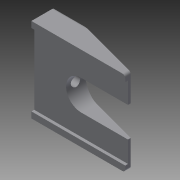
# Autodesk Inventor part: Sliding Block
Saved by Autodesk Inventor 2015 SP2 (Build 190223200, 223)
## iProperties
Created: 2015-12-04
Part Number: Sliding Block
Material: Generic
Document SubType Name: Sheet Metal
Designer: KC-019
Density: 1 g/cm^3
Sheet Metal Rule: Default_mm
Appearance: Default
Author: KC-019
Autodesk Inventor part; units mm, degrees
ref_plane "YZ Plane" through (0, 0, 0) normal (1, 0, 0) x (0, 1, 0)
ref_plane "XZ Plane" through (0, 0, 0) normal (0, 1, 0) x (-1, 0, 0)
ref_plane "XY Plane" through (0, 0, 0) normal (0, 0, 1) x (1, 0, 0)
sketch "Sketch1" plane through (0, 0, 0) normal (0, 1, 0) x (-1, 0, 0)
  arc A0 (0, -16) -> (0, 16) centre (0, 0) ccw
  line L0 (0, 16) -> (-50, 16)
  line L1 (-50, 16) -> (-50, -16)
  line L2 (-50, -16) -> (0, -16)
  line L3 (-50, 0) -> (-50, -45)
  line L4 (-50, -45) -> (-50, 45)
  line L5 (-50, 45) -> (50, 45)
  line L6 (50, 45) -> (50, -45)
  line L7 (50, -45) -> (-50, -45)
  dimension "d1" = 32
  dimension "d2" = 50
  dimension "d3" = 45
  dimension "d4" = 90
  dimension "d5" = 100
  constraints: 16 end point, 4 perpendicular, 2 point on circle, 2 point on line, 2 tangent, 1 centre point, 1 horizontal, 1 midpoint
  measures "d1" diameter of A0
  measures "d2" distance of L0.start L0.end
  measures "d3" distance of L3.start L3.end
  measures "d4" distance of L3.end L4.end
  measures "d5" distance of L4.end L5.end
extrude "Extrusion1" add sketch "Sketch1" along normal blind 25 contours A0 L0 L4 L5 L6 L7 L3 L2
sketch "Sketch2" plane through (-50, 0, 45) normal (0, 0, 1) x (1, 0, 0)
  line L0 (0, 0) -> (100, 0)
  line L1 (50, 0) -> (100, 0) projected
  line L2 (100, 0) -> (100, 6)
  line L3 (100, 0) -> (100, 25) projected
  line L4 (0, 0) -> (0, 25)
  line L5 (0, 25) -> (29.091, 25)
  line L6 (0, 25) -> (100, 25) projected
  line L7 (29.091, 25) -> (100, 6)
  line L8 (29.091, 25) -> (100, 25)
  line L9 (100, 25) -> (100, 6)
  dimension "d8" = 6
  constraints: 14 end point, 2 perpendicular, 2 point on line, 1 collinear, 1 vertical
  measures "d8" distance of L0.end L2.end
extrude "Extrusion2" cut sketch "Sketch2" against normal through all contours L6 L3 L7
sketch "Sketch3" plane through (50, 0, 45) normal (1, 0, 0) x (0, 0, -1)
  line L0 (45, 0) -> (83.5, 0)
  line L1 (90, 0) -> (0, 0) projected
  line L2 (45, 0) -> (6.5, 0)
  line L3 (0, 0) -> (29, 0) projected
  line L4 (83.5, 0) -> (83.5, 3)
  line L5 (83.5, 3) -> (6.5, 3)
  line L6 (6.5, 0) -> (6.5, 3)
  dimension "d12" = 38.5
  dimension "d13" = 38.5
  dimension "d14" = 3
  constraints: 10 end point, 2 point on line, 1 parallel, 1 perpendicular, 1 vertical
  measures "d12" distance of L0.start L0.end
  measures "d13" distance of L0.start L2.end
  measures "d14" distance of L0.end L4.end
extrude "Extrusion3" cut sketch "Sketch3" against normal through all
sketch "Sketch4" plane through (-50, 0, 45) normal (-1, 0, 0) x (0, 0, 1)
  line L0 (-45, 0) -> (-45, 13)
  circle A0 centre (-45, 13) radius 5
  dimension "d17" = 13
  dimension "d18" = 10
  constraints: 2 end point, 1 centre point, 1 coincident, 1 vertical
  measures "d17" distance of L0.start L0.end
  measures "d18" diameter of A0
extrude "Extrusion4" cut sketch "Sketch4" against normal through all
fillet "Fillet1" radius 3 4 edges at (-35.4545, 25, 45) (-35.4545, 25, -45) (50, 3, 45) (50, 3, -45)
equation "\"BendRadius\" = Thickness"
equation "\"BendReliefWidth\" = Thickness"
equation "\"BendReliefDepth\" = 0.5 * Thickness"
equation "\"CornerReliefSize\" = 4 * Thickness"
equation "\"MinimumRemnant\" = 2 * Thickness"
equation "\"TransitionRadius\" = BendRadius"
equation "\"JacobiRadiusSize\" = BendRadius"
equation "\"GapSize\" = Thickness"
equation "\"Thickness\" = 0.5"
body "Solid1"
